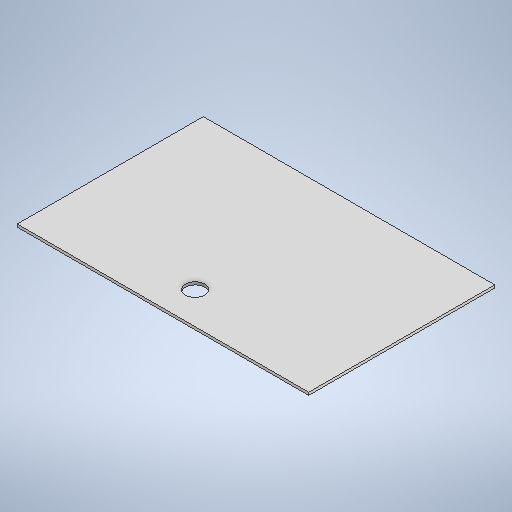
# Autodesk Inventor part: scina_prawa
Saved by Autodesk Inventor 2026.2 (Build 302298010, 298A)
## iProperties
Created: 2026-04-29
Part Number: scina_prawa
Material: Ogólny
Document SubType Name: Modeling
Designer: Patryk
Density: 1 g/cm^3
Appearance: Domyślna
Author: Patryk
Autodesk Inventor part; units mm, degrees
ref_plane "YZ Plane" through (0, 0, 0) normal (1, 0, 0) x (0, 1, 0)
ref_plane "XZ Plane" through (0, 0, 0) normal (0, 1, 0) x (-1, 0, 0)
ref_plane "XY Plane" through (0, 0, 0) normal (0, 0, 1) x (1, 0, 0)
sketch "Szkic1" plane through (0, 0, 0) normal (0, 1, 0) x (-1, 0, 0)
  line L0 (-159, -101.5) -> (159, -101.5)
  line L1 (159, -101.5) -> (159, 101.5)
  line L2 (159, 101.5) -> (-159, 101.5)
  line L3 (-159, 101.5) -> (-159, -101.5)
  line L4 (-159, -101.5) -> (159, 101.5) construction
  line L5 (159, -101.5) -> (-159, 101.5) construction
  circle A0 centre (0, 66.5) radius 10.5
  point P0 (0, 0)
  dimension "d0" = 318
  dimension "d1" = 203
  dimension "d2" = 21
  dimension "d3" = 35
  dimension "d4" = 159
  constraints: 12 end point, 2 midpoint, 2 parallel, 1 centre point, 1 horizontal, 1 perpendicular
  measures "d0" distance of L2.end L1.end
  measures "d1" distance of L1.end L0.end
  measures "d2" diameter of A0
  measures "d3" distance from line of L2 A0.centre
  measures "d4" distance from line of L1 A0.centre
extrude "Wyciągnięcie proste1" add sketch "Szkic1" along normal mid plane 3
